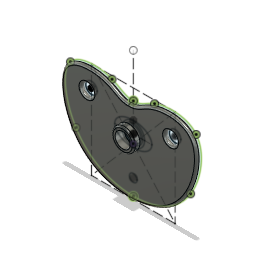
Shield (Autodesk Fusion 360 design; units mm, degrees)
Autodesk Fusion 360 part; units mm, degrees
note: some values were not read from the file. Chosen so that the rebuilt part matches the saved one: which face or edge a step refers to.
sketch "Sketch1" plane through (0, 0, 0) normal (0, 0, 1) x (1, 0, 0)
  line L0 (0, 0) -> (0, 53.2713) construction
  spline S0 degree 5 poles (0, 24.3725) (-0.8697, 24.3599) (-2.5208, 24.4619) (-4.7326, 24.9961) (-7.3449, 26.3669) (-10.9471, 28.6062) (-15.7271, 30.6761) (-21.8521, 31.9781) (-28.644, 32.1222) (-35.0866, 30.8696) (-40.1907, 28.1177) (-43.3626, 23.8741) (-44.9293, 18.2314) (-45.0514, 11.5279) (-43.8678, 4.2293) (-41.473, -3.1386) (-37.9558, -10.0737) (-33.4141, -16.1748) (-27.9796, -21.2217) (-21.7982, -25.1271) (-15.0131, -27.8943) (-9.2009, -29.2397) (-4.6651, -29.7883) (-1.5673, -29.9539) (0, -29.9867) knots 0 0 0 0 0 0 0.05 0.1 0.15 0.2 0.25 0.3 0.35 0.4 0.45 0.5 0.55 0.6 0.65 0.7 0.75 0.8 0.85 0.9 0.95 1 1 1 1 1 1
  line L1 (-10.4969, -29.7672) -> (10.4969, -30.2062)
  line L2 (10.131, 24.5188) -> (-10.131, 24.2261)
  spline S1 degree 5 poles (0, 24.3725) (0.8697, 24.3599) (2.5208, 24.4619) (4.7326, 24.9961) (7.3449, 26.3669) (10.9471, 28.6062) (15.7271, 30.6761) (21.8521, 31.9781) (28.644, 32.1222) (35.0866, 30.8696) (40.1907, 28.1177) (43.3626, 23.8741) (44.9293, 18.2314) (45.0514, 11.5279) (43.8678, 4.2293) (41.473, -3.1386) (37.9558, -10.0737) (33.4141, -16.1748) (27.9796, -21.2217) (21.7982, -25.1271) (15.0131, -27.8943) (9.2009, -29.2397) (4.6651, -29.7883) (1.5673, -29.9539) (0, -29.9867) knots 0 0 0 0 0 0 0.05 0.1 0.15 0.2 0.25 0.3 0.35 0.4 0.45 0.5 0.55 0.6 0.65 0.7 0.75 0.8 0.85 0.9 0.95 1 1 1 1 1 1
  line L3 (-10.131, 24.5188) -> (10.131, 24.2261)
  line L4 (10.4969, -29.7672) -> (-10.4969, -30.2062)
  line L5 (-36.675, 31.9753) -> (-46.186, 19.9768)
  line L6 (36.675, 31.9753) -> (46.186, 19.9768)
  line L7 (-27.5527, 31.8452) -> (27.5527, 31.8452) construction
  line L8 (27.5527, 31.8452) -> (27.5527, -31.8452) construction
  line L9 (27.5527, -31.8452) -> (-27.5527, -31.8452) construction
  line L10 (-27.5527, -31.8452) -> (-27.5527, 31.8452) construction
  line L11 (-27.5527, 31.8452) -> (27.5527, -31.8452) construction
  line L12 (27.5527, 31.8452) -> (-27.5527, -31.8452) construction
  circle A0 centre (-27.5527, 18.0952) radius 3.75
  circle A1 centre (27.5527, 18.0952) radius 3.75
  ellipse E0 centre (0, 5.4975) end of major axis (12.2, 5.4975) minor radius 7.875
  line L13 (-12.2, 5.4975) -> (12.2, 5.4975)
  line L14 (0, -2.3775) -> (0, 13.3725)
  circle A2 centre (0, 5.4975) radius 5
  circle A3 centre (0, 5.4975) radius 7.41
  circle A4 centre (0, -19.5025) radius 2.5
  circle A5 centre (0, 5.4975) radius 6.07
  point P0 (-14.0123, 29.7864)
  point P1 (-41.4305, 25.976)
  point P2 (-37.7899, -9.7209)
  point P3 (14.0123, 29.7864)
  point P4 (41.4305, 25.976)
  point P5 (37.7899, -9.7209)
  point P6 (0, 13.3725)
  dimension "d1" = 7.5
  dimension "d2" = 13.75
  dimension "d3" = 24.4
  dimension "d4" = 15.75
  dimension "d5" = 11
  dimension "d15" = 10
  dimension "d16" = 2.41
  dimension "d81" = 5
  dimension "d82" = 25
  dimension "d89" = 12.14
  dimension "d6" = 55.1055
  constraint coincident L0.start origin
  constraint vertical L0
  constraint midpoint S0.end L1
  constraint midpoint S0.start L2
  constraint symmetric L0 S0.start S1.start
  constraint symmetric L0 P0 P3
  constraint symmetric L0 P1 P4
  constraint symmetric L0 P2 P5
  constraint symmetric L0 S0.end S1.end
  constraint symmetric L0 L1.start L4.start
  constraint symmetric L0 L1.end L4.end
  constraint symmetric L0 L2.start L3.start
  constraint symmetric L0 L2.end L3.end
  constraint midpoint P1 L5
  constraint symmetric L0 L5.start L6.start
  constraint symmetric L0 L5.end L6.end
  constraint midpoint P4 L6
  constraint horizontal L7
  constraint perpendicular L7 L8
  constraint parallel L7 L9
  constraint parallel L8 L10
  constraint coincident L11 L0.start
  constraint coincident L12 L0.start
  constraint coincident S0 L7.start
  constraint coincident L10 A0.centre
  constraint symmetric L0 A0 A1
  constraint coincident E0 L13.start
  constraint coincident E0 L13.end
  constraint coincident E0 L14.start
  constraint coincident E0 P6
  constraint coincident L0 E0.centre
  constraint perpendicular L0 L13
  constraint coincident P6 L14.end
  constraint concentric E0 A2
  constraint concentric A2 A3
  constraint vertical E0.centre A4.centre
  constraint concentric E0 A5
  measures "d1" diameter of A0
  measures "d2" distance of L7.start A0.centre
  measures "d3" distance of E0
  measures "d5" distance of S0.start P6
  measures "d15" diameter of A2
  measures "d16" distance of A2 A3
  measures "d81" diameter of A4
  measures "d82" distance of E0.centre A4.centre
  measures "d89" diameter of A5
  measures "d6" distance of L8.end L9.end
extrude "Extrude6" add sketch "Sketch1" along normal blind 3 contours S0 S1 | E0 L13 L14 A3 | E0 L13 L14 A3 | E0 L13 L14 A3 | E0 L13 L14 A3 | A4
extrude "Extrude7" add sketch "Sketch1" along normal blind 7 contours L13 L14 A3 A5 | L13 L14 A3 A5 | L13 L14 A3 A5 | L13 L14 A3 A5 | L13 L14 A2 A5 | L13 L14 A2 A5 | L13 L14 A2 A5 | L13 L14 A2 A5
extrude "Extrude8" cut sketch "Sketch1" along normal blind 0.9 contours L13 L14 A2 A5 | L13 L14 A2 A5 | L13 L14 A2 A5 | L13 L14 A2 A5
fillet "Fillet4" radius 1 1 edges at (-6.9085, 2.8179, 7)
fillet "Fillet5" radius 1.5 4 faces at (39.2816, -7.1026, 2) (31.2981, 17.9083, 2) (-23.8074, 17.9083, 2) (-0.4797, 24.3734, 2.5417)
equation "d2 = 10 mm + ( ( 7.5 / 2 ) * 1 mm )"
equation "Thickness = 3 mm"
equation "d8 = Thickness"
equation "d10 = Thickness + ProtrusionExtra"
equation "ProtrusionExtra = 4 mm"
